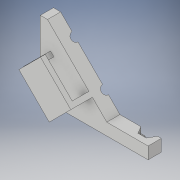
# Autodesk Inventor part: e27_Holder_v2
Saved by Autodesk Inventor 2019 (Build 230136000, 136)
## iProperties
Created: 2019-05-10
Part Number: e27_Holder_v2
Material: Generic
Document SubType Name: Modeling
Designer: Daniel
Density: 1 g/cm^3
Appearance: Default
Author: Daniel
## iProperties of the stored document e27_Holder_v2_3DPrint.ipt
Created: 2019-05-10
Part Number: e27_Holder_v2_3DPrint
Material: Generic
Document SubType Name: Modeling
Designer: Daniel
Density: 1 g/cm^3
Appearance: Default
Author: Daniel
Autodesk Inventor part; units mm, degrees
ref_plane "YZ Plane" through (0, 0, 0) normal (1, 0, 0) x (0, 1, 0)
ref_plane "XZ Plane" through (0, 0, 0) normal (0, 1, 0) x (-1, 0, 0)
ref_plane "XY Plane" through (0, 0, 0) normal (0, 0, 1) x (1, 0, 0)
sketch "Base" plane through (0, 0, 0) normal (0, 0, 1) x (1, 0, 0)
  line L0 (0, 0) -> (-24.7487, 24.7487)
  line L1 (0, 0) -> (35, 0) construction
  line L2 (-24.7487, 24.7487) -> (-24.7487, 0)
  line L3 (-24.7487, 0) -> (0, 0)
  line L4 (-24.7487, 24.7487) -> (-27.7487, 24.7487)
  line L5 (-27.7487, 24.7487) -> (-27.7487, 0)
  line L6 (-27.7487, 0) -> (-24.7487, 0)
  line L7 (-24.7487, 0) -> (-24.7487, 24.7487)
  line L8 (-27.7487, 0) -> (17.2513, 0)
  line L9 (17.2513, 0) -> (17.2513, -5)
  line L10 (17.2513, -5) -> (-27.7487, -5)
  line L11 (-27.7487, -5) -> (-27.7487, 0)
  line L12 (3, 15.0208) -> (-9.7279, 27.7487)
  line L13 (-9.7279, 27.7487) -> (-27.7487, 9.7279)
  line L14 (-27.7487, 9.7279) -> (-15.0208, -3)
  line L15 (-15.0208, -3) -> (3, 15.0208)
  line L16 (3, 15.0208) -> (-27.7487, 9.7279) construction
  line L17 (-9.7279, 27.7487) -> (-15.0208, -3) construction
  line L18 (-24.9203, 9.7279) -> (-9.7279, 24.9203)
  line L19 (-9.7279, 24.9203) -> (0.1716, 15.0208)
  line L20 (0.1716, 15.0208) -> (-15.0208, -0.1716)
  line L21 (-15.0208, -0.1716) -> (-24.9203, 9.7279)
  line L22 (-18.7383, 18.7383) -> (-17.3241, 17.3241)
  line L23 (-7.4246, 7.4246) -> (-6.0104, 6.0104)
  line L24 (-27.7487, 9.7279) -> (-23.5061, 13.9706)
  line L25 (-23.5061, 13.9706) -> (-22.0919, 12.5564)
  line L26 (-22.0919, 12.5564) -> (-26.3345, 8.3137)
  line L27 (-26.3345, 8.3137) -> (-27.7487, 9.7279)
  line L28 (-23.5061, 5.4853) -> (-19.2635, 1.2426)
  line L29 (-16.435, 4.0711) -> (-23.5061, 5.4853) construction
  line L30 (-20.6777, 8.3137) -> (-19.2635, 1.2426) construction
  line L31 (-6.0104, 6.0104) -> (-7.4246, 7.4246)
  line L32 (-7.4246, 7.4246) -> (-16.435, -1.5858)
  line L33 (-16.435, -1.5858) -> (-15.0208, -3)
  line L34 (-15.0208, -3) -> (-6.0104, 6.0104)
  line L35 (-15.0208, -0.1716) -> (-17.8492, 2.6569)
  line L36 (-17.8492, 2.6569) -> (-19.2635, 1.2426)
  line L37 (-19.2635, 1.2426) -> (-16.435, -1.5858)
  line L38 (-16.435, -1.5858) -> (-15.0208, -0.1716)
  line L39 (-26.3345, 8.3137) -> (-23.5061, 5.4853)
  line L40 (-23.5061, 5.4853) -> (-22.0919, 6.8995)
  line L41 (-22.0919, 6.8995) -> (-24.9203, 9.7279)
  line L42 (-24.9203, 9.7279) -> (-26.3345, 8.3137)
  point P0 (-12.3744, 12.3744)
  point P1 (-19.9706, 4.7782)
  dimension "d0" = 35
  dimension "d1" = 135
  dimension "d2" = 3
  dimension "d3" = 45
  dimension "d4" = 5
  dimension "d5" = 18
  dimension "d6" = 2
  dimension "d7" = 6
  constraints: 86 end point, 16 parallel, 10 midpoint, 10 perpendicular, 3 horizontal, 2 point on line, 1 collinear, 1 equal length, 1 vertical, 3 other
  measures "d0" distance of L0.start L0.end
  measures "d1" angle of L1 L0
  measures "d2" distance of L6.end L5.end
  measures "d3" distance of L9.end L10.end
  measures "d4" distance of L8.end L9.end
  measures "d5" distance of L12.start L12.end
  measures "d6" distance between parallel lines of L13 L18
  measures "d7" distance of L13.end L24.end
extrude "Extrusion1" add sketch "Base" along normal blind 5.5 contours L3 L15 L0 | L8 L9 L10 L11 L6 L3 L14 L15 | L15 L3 L20 L0 | L15 L14 L32 L20 L3 | L20 L3 L21 L2 L18 L0 | L20 L21 L3 | L18 L25 L13 L0 | L21 L32 L14 L3 | L3 L14 L36 L21 | L13 L2 L0 | L18 L2 L13 L25 | L3 L2 L14 | L36 L14 L40 L21 | L5 L14 L2 L6 | L2 L13 L5 L4 | L18 L26 L14 L13 L2 | L2 L21 L18 | L40 L14 L2 L21 | L2 L14 L26 L21
extrude "Extrusion2" add sketch "Base" along normal blind 12.5 contours L15 L3 L20 L0 | L15 L14 L32 L20 L3 | L21 L32 L14 L3 | L3 L14 L36 L21 | L18 L2 L13 L25 | L18 L26 L14 L13 L2 | L40 L14 L2 L21 | L2 L14 L26 L21
sketch "TouchProtection" plane through (0, 0, 12.5) normal (0, 0, 1) x (1, 0, 0)
  line L0 (-6.0104, 6.0104) -> (-15.0208, -3) projected
  line L1 (-6.0104, 6.0104) -> (-15.0208, -3)
  line L2 (-15.0208, -3) -> (-27.6905, 9.6697)
  line L3 (-27.6905, 9.6697) -> (-18.6801, 18.6801)
  line L4 (-18.6801, 18.6801) -> (-6.0104, 6.0104)
  point P0 (0, 0)
  constraints: 8 end point, 3 equal length, 1 perpendicular
extrude "Extrusion3" add sketch "TouchProtection" along normal blind 2
sketch "MountingHolesBottom" plane through (-27.7487, -5, 0) normal (0, -1, 0) x (1, 0, 0)
  line L0 (0, 0) -> (5, 0)
  line L1 (45, 0) -> (40, 0)
  circle A0 centre (5, 0) radius 1.75
  circle A1 centre (40, 0) radius 1.75
  line L2 (5, 0) -> (5, 3)
  line L3 (5, 0) -> (8, 0) construction
  line L4 (6.7321, 3) -> (8.4641, 0)
  line L5 (8.4641, 0) -> (6.7321, -3)
  line L6 (6.7321, -3) -> (3.2679, -3)
  line L7 (3.2679, -3) -> (1.5359, 0)
  line L8 (1.5359, 0) -> (3.2679, 3)
  line L9 (3.2679, 3) -> (6.7321, 3)
  line L10 (40, 0) -> (40, 3)
  line L11 (41.7321, 3) -> (43.4641, 0)
  line L12 (43.4641, 0) -> (41.7321, -3)
  line L13 (41.7321, -3) -> (38.2679, -3)
  line L14 (38.2679, -3) -> (36.5359, 0)
  line L15 (36.5359, 0) -> (38.2679, 3)
  line L16 (38.2679, 3) -> (41.7321, 3)
  line L17 (1.5359, 0) -> (43.4641, 0)
  point P0 (27.7487, 0)
  dimension "d15" = 5
  dimension "d16" = 5
  dimension "d17" = 3.5
  dimension "d18" = 3.5
  dimension "d19" = 3
  dimension "d20" = 90
  dimension "d21" = 3
  constraints: 36 end point, 4 coincident, 2 centre point, 2 midpoint, 1 horizontal, 1 perpendicular, 1 vertical, 26 other
  measures "d15" distance of L0.start L0.end
  measures "d16" distance of L1.start L1.end
  measures "d17" diameter of A0
  measures "d18" diameter of A1
  measures "d19" distance of L2.start L2.end
  measures "d20" angle of L3 L2
  measures "d21" distance of L10.start L10.end
extrude "Extrusion4" cut sketch "MountingHolesBottom" against normal blind 10 contours A0 L2 L0 | L0 L17 A0 | L2 A0 L17 | L17 L1 A1 | A1 L10 L17 | A1 L1 L10
extrude "Extrusion5" cut sketch "MountingHolesBottom" against normal blind 6 contours L8 L9 L2 A0 L0 | L0 A0 L17 L5 L6 L7 | L15 L16 L10 A1 L17 | L17 A1 L1 L12 L13 L14 | L2 L9 L4 L17 A0 | L16 L11 L1 A1 L10
extrude "Extrusion6" add sketch "MountingHolesBottom" against normal blind 2.5 contours L8 L9 L2 A0 L0 | L0 A0 L17 L5 L6 L7 | L15 L16 L10 A1 L17 | L17 A1 L1 L12 L13 L14 | L2 L9 L4 L17 A0 | L16 L11 L1 A1 L10
sketch "MountingHolesE27" plane through (0, 0, 0) normal (0.7071, 0.7071, 0) x (-0.7071, 0.7071, 0)
  line L0 (0, 0) -> (0, 5.5) projected
  line L1 (0, 0) -> (8.5, 0)
  line L2 (0, 0) -> (35, 0) projected
  line L3 (8.5, 0) -> (26.5, 0)
  circle A0 centre (8.5, 0) radius 1.75
  circle A1 centre (26.5, 0) radius 1.75
  line L4 (8.5, 0) -> (8.5, 3)
  line L5 (26.5, 0) -> (26.5, 3)
  line L6 (26.5, 0) -> (29.5, 0) construction
  line L7 (28.2321, 3) -> (29.9641, 0)
  line L8 (29.9641, 0) -> (28.2321, -3)
  line L9 (28.2321, -3) -> (24.7679, -3)
  line L10 (24.7679, -3) -> (23.0359, 0)
  line L11 (23.0359, 0) -> (24.7679, 3)
  line L12 (24.7679, 3) -> (28.2321, 3)
  line L13 (10.2321, 3) -> (11.9641, 0)
  line L14 (11.9641, 0) -> (10.2321, -3)
  line L15 (10.2321, -3) -> (6.7679, -3)
  line L16 (6.7679, -3) -> (5.0359, 0)
  line L17 (5.0359, 0) -> (6.7679, 3)
  line L18 (6.7679, 3) -> (10.2321, 3)
  dimension "d30" = 8.5
  dimension "d31" = 18
  dimension "d32" = 180
  dimension "d33" = 3.5
  dimension "d34" = 3.5
  dimension "d35" = 3
  dimension "d36" = 3
  dimension "d37" = 90
  constraints: 34 end point, 4 coincident, 2 centre point, 2 midpoint, 2 vertical, 1 collinear, 1 horizontal, 1 perpendicular, 1 point on line, 26 other
  measures "d30" distance of L0.start L1.end
  measures "d31" distance of L1.end L3.end
  measures "d32" angle of L3 L1
  measures "d33" diameter of A0
  measures "d34" diameter of A1
  measures "d35" distance of L4.start L4.end
  measures "d36" distance of L5.start L5.end
  measures "d37" angle of L6 L5
extrude "Extrusion8" cut sketch "MountingHolesE27" against normal blind 10 contours A0 L4 L1 | L1 L2 A0 | L4 A0 L2 | A1 L5 L2 | L2 A1 | L5 A1 L2
extrude "Extrusion9" cut sketch "MountingHolesE27" against normal blind 7 contours L17 L18 L4 A0 L1 | L1 A0 L2 L14 L15 L16 | L11 L12 L5 A1 L2 | L2 A1 L8 L9 L10 | L4 L18 L13 L2 A0 | L5 L12 L7 L2 A1
extrude "Extrusion10" add sketch "MountingHolesE27" against normal blind 4 contours L17 L18 L4 A0 L1 | L1 A0 L2 L14 L15 L16 | L11 L12 L5 A1 L2 | L2 A1 L8 L9 L10 | L4 L18 L13 L2 A0 | L5 L12 L7 L2 A1
sketch "Sketch7" plane through (0, 0, 0) normal (0, 0, -1) x (-1, 0, 0)
  line L0 (-17.2513, -5) -> (-17.2513, 0) projected
  line L1 (24.7487, 24.7487) -> (27.7487, 24.7487) projected
  line L2 (-17.2513, -5) -> (27.7487, -5)
  line L3 (27.7487, -5) -> (27.7487, 24.7487)
  line L4 (27.7487, 24.7487) -> (-17.2513, 24.7487)
  line L5 (-17.2513, 24.7487) -> (-17.2513, -5)
  point P0 (0, 0)
  constraints: 8 end point, 2 parallel, 1 horizontal, 1 perpendicular
extrude "Extrusion11" cut sketch "Sketch7" along normal blind 21.25
sketch "Sketch8" plane through (0, 0, 0) normal (0, 0, -1) x (-1, 0, 0)
  line L0 (7.2478, 7.2478) -> (17.5009, 17.5009) projected
  line L1 (12.3744, 12.3744) -> (13.0815, 11.6673)
  line L2 (12.3744, 12.3744) -> (13.3744, 12.3744) construction
  line L3 (13.0815, 11.6673) -> (15.9099, 8.8388)
  line L4 (18.4555, 5.7276) -> (12.7986, 11.3844)
  line L5 (12.7986, 11.3844) -> (13.3643, 11.9501)
  line L6 (13.3643, 11.9501) -> (19.0212, 6.2933)
  line L7 (19.0212, 6.2933) -> (18.4555, 5.7276)
  line L8 (18.4555, 5.7276) -> (13.3643, 11.9501) construction
  line L9 (12.7986, 11.3844) -> (19.0212, 6.2933) construction
  line L10 (-10.5258, -5.0105) -> (-2.5258, -5.0105)
  line L11 (20.9987, -5) -> (-10.5013, -5) projected
  line L12 (-10.5258, -5.0105) -> (-2.5258, -5.0105) construction
  line L13 (-2.5258, -5.0105) -> (-2.5258, -2.5105)
  line L14 (-6.5258, -2.1105) -> (1.4742, -2.1105)
  line L15 (1.4742, -2.1105) -> (1.4742, -2.9105)
  line L16 (1.4742, -2.9105) -> (-6.5258, -2.9105)
  line L17 (-6.5258, -2.9105) -> (-6.5258, -2.1105)
  line L18 (-6.5258, -2.1105) -> (1.4742, -2.9105) construction
  line L19 (1.4742, -2.1105) -> (-6.5258, -2.9105) construction
  point P0 (0, 0)
  dimension "d46" = 1
  dimension "d47" = 45
  dimension "d48" = 4
  dimension "d49" = 0.8
  dimension "d50" = 8
  dimension "d51" = 0
  dimension "d52" = 2.5
  dimension "d53" = 8
  dimension "d54" = 0.8
  constraints: 36 end point, 6 parallel, 5 midpoint, 4 perpendicular, 3 horizontal, 2 equal length
  measures "d46" distance of L1.start L1.end
  measures "d47" angle of L1 L2
  measures "d48" distance of L1.end L3.end
  measures "d49" distance of L4.end L5.end
  measures "d50" distance of L10.start L10.end
  measures "d51" distance between parallel lines of L10 L12
  measures "d52" distance of L10.end L13.end
  measures "d53" distance of L15.end L16.end
  measures "d54" distance of L14.end L15.end
extrude "Extrusion12" cut sketch "Sketch8" against normal blind 4
body "Solid1"
